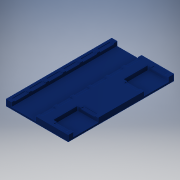
# Autodesk Inventor part: Assembly Plate
Saved by Autodesk Inventor 2019.4 (Build 234330000, 330)
## iProperties
Created: 2021-01-11
Part Number: Assembly Plate
Material: Aluminum, Anodized Blue
Document SubType Name: Modeling
Designer: caleb
Density: 2.7 g/cm^3
Appearance: Anodized - Blue
Author: caleb
Autodesk Inventor part; units mm, degrees
ref_plane "YZ Plane" through (0, 0, 0) normal (1, 0, 0) x (0, 1, 0)
ref_plane "XZ Plane" through (0, 0, 0) normal (0, 1, 0) x (-1, 0, 0)
ref_plane "XY Plane" through (0, 0, 0) normal (0, 0, 1) x (1, 0, 0)
sketch "Sketch1" plane through (0, 0, 0) normal (0, 1, 0) x (-1, 0, 0)
  line L0 (-63.5, 107.95) -> (63.5, 107.95)
  line L1 (63.5, 107.95) -> (63.5, -107.95)
  line L2 (63.5, -107.95) -> (-63.5, -107.95)
  line L3 (-63.5, -107.95) -> (-63.5, 107.95)
  line L4 (-63.5, 107.95) -> (63.5, -107.95) construction
  line L5 (63.5, 107.95) -> (-63.5, -107.95) construction
  point P0 (0, 0)
  dimension "d0" = 127
  dimension "d1" = 215.9
  constraints: 12 end point, 2 midpoint, 2 parallel, 1 horizontal, 1 perpendicular
  measures "d0" distance of L1.end L2.end
  measures "d1" distance of L0.end L1.end
extrude "Extrusion1" add sketch "Sketch1" along normal blind 12.7
sketch "Sketch8" plane through (0, 12.7, 0) normal (0, 1, 0) x (1, 0, 0)
  line L0 (-63.5, -107.95) -> (63.5, -107.95) projected
  line L1 (63.5, 107.95) -> (-63.5, 107.95) projected
  line L2 (-63.5, 107.95) -> (-63.5, -107.95) projected
  line L3 (63.5, -107.95) -> (63.5, 107.95) projected
  line L4 (-52.5, -107.95) -> (-2.5, -107.95)
  line L5 (-2.5, -107.95) -> (-2.5, 107.95)
  line L6 (-2.5, 107.95) -> (-52.5, 107.95)
  line L7 (-52.5, 107.95) -> (-52.5, -107.95)
  point P0 (0, 0)
  dimension "d91" = 11
  dimension "d92" = 50
  constraints: 8 end point, 2 parallel, 2 point on line, 1 horizontal, 1 perpendicular
  measures "d91" distance between parallel lines of L2 L7
  measures "d92" distance between parallel lines of L7 L5
extrude "Extrusion7" cut sketch "Sketch8" against normal blind 9 contours L7 L1 L5 L0
sketch "Sketch9" plane through (0, 12.7, 0) normal (0, 1, 0) x (1, 0, 0)
  line L0 (-63.5, -107.95) -> (-52.5, -107.95) projected
  line L1 (-63.5, 107.95) -> (-63.5, -107.95) projected
  line L2 (-52.5, -107.95) -> (-52.5, 107.95) projected
  line L3 (-52.5, -100.922) -> (-59, -100.922)
  line L4 (-59, -100.922) -> (-59, -74.122)
  line L5 (-58, -73.122) -> (-52.5, -73.122)
  line L6 (-52.5, -73.122) -> (-52.5, -100.922)
  circle A0 centre (-59, -100.922) radius 1
  line L7 (-2.5, 107.95) -> (-2.5, -107.95) projected
  line L8 (-2.5, -107.95) -> (63.5, -107.95) projected
  line L9 (-2.5, -100.922) -> (3, -100.922)
  line L10 (4, -99.922) -> (4, -74.122)
  line L11 (3, -73.122) -> (-2.5, -73.122)
  line L12 (-2.5, -73.122) -> (-2.5, -100.922)
  arc A1 (-58, -73.122) -> (-59, -74.122) centre (-58, -74.122) ccw
  arc A2 (4, -74.122) -> (3, -73.122) centre (3, -74.122) ccw
  arc A3 (3, -100.922) -> (4, -99.922) centre (3, -99.922) ccw
  arc A4 (4, -39.294) -> (3, -38.294) centre (3, -39.294) ccw
  line L13 (-2.5, -38.294) -> (-2.5, -66.094)
  line L14 (4, -65.094) -> (4, -39.294)
  line L15 (-2.5, -66.094) -> (3, -66.094)
  arc A5 (3, -66.094) -> (4, -65.094) centre (3, -65.094) ccw
  line L16 (3, -38.294) -> (-2.5, -38.294)
  line L17 (-52.5, -38.294) -> (-52.5, -66.094)
  line L18 (-58, -38.294) -> (-52.5, -38.294)
  arc A6 (-58, -38.294) -> (-59, -39.294) centre (-58, -39.294) ccw
  line L19 (-59, -66.094) -> (-59, -39.294)
  line L20 (-52.5, -66.094) -> (-59, -66.094)
  circle A7 centre (-59, -66.094) radius 1
  arc A8 (4, -4.466) -> (3, -3.466) centre (3, -4.466) ccw
  line L21 (-2.5, -3.466) -> (-2.5, -31.266)
  line L22 (4, -30.266) -> (4, -4.466)
  line L23 (-2.5, -31.266) -> (3, -31.266)
  arc A9 (3, -31.266) -> (4, -30.266) centre (3, -30.266) ccw
  line L24 (3, -3.466) -> (-2.5, -3.466)
  line L25 (-52.5, -3.466) -> (-52.5, -31.266)
  line L26 (-58, -3.466) -> (-52.5, -3.466)
  arc A10 (-58, -3.466) -> (-59, -4.466) centre (-58, -4.466) ccw
  line L27 (-59, -31.266) -> (-59, -4.466)
  line L28 (-52.5, -31.266) -> (-59, -31.266)
  circle A11 centre (-59, -31.266) radius 1
  arc A12 (4, 30.362) -> (3, 31.362) centre (3, 30.362) ccw
  line L29 (-2.5, 31.362) -> (-2.5, 3.562)
  line L30 (4, 4.562) -> (4, 30.362)
  line L31 (-2.5, 3.562) -> (3, 3.562)
  arc A13 (3, 3.562) -> (4, 4.562) centre (3, 4.562) ccw
  line L32 (3, 31.362) -> (-2.5, 31.362)
  line L33 (-52.5, 31.362) -> (-52.5, 3.562)
  line L34 (-58, 31.362) -> (-52.5, 31.362)
  arc A14 (-58, 31.362) -> (-59, 30.362) centre (-58, 30.362) ccw
  line L35 (-59, 3.562) -> (-59, 30.362)
  line L36 (-52.5, 3.562) -> (-59, 3.562)
  circle A15 centre (-59, 3.562) radius 1
  arc A16 (4, 65.19) -> (3, 66.19) centre (3, 65.19) ccw
  line L37 (-2.5, 66.19) -> (-2.5, 38.39)
  line L38 (4, 39.39) -> (4, 65.19)
  line L39 (-2.5, 38.39) -> (3, 38.39)
  arc A17 (3, 38.39) -> (4, 39.39) centre (3, 39.39) ccw
  line L40 (3, 66.19) -> (-2.5, 66.19)
  line L41 (-52.5, 66.19) -> (-52.5, 38.39)
  line L42 (-58, 66.19) -> (-52.5, 66.19)
  arc A18 (-58, 66.19) -> (-59, 65.19) centre (-58, 65.19) ccw
  line L43 (-59, 38.39) -> (-59, 65.19)
  line L44 (-52.5, 38.39) -> (-59, 38.39)
  circle A19 centre (-59, 38.39) radius 1
  arc A20 (4, 100.018) -> (3, 101.018) centre (3, 100.018) ccw
  line L45 (-2.5, 101.018) -> (-2.5, 73.218)
  line L46 (4, 74.218) -> (4, 100.018)
  line L47 (-2.5, 73.218) -> (3, 73.218)
  arc A21 (3, 73.218) -> (4, 74.218) centre (3, 74.218) ccw
  line L48 (3, 101.018) -> (-2.5, 101.018)
  line L49 (-52.5, 101.018) -> (-52.5, 73.218)
  line L50 (-58, 101.018) -> (-52.5, 101.018)
  arc A22 (-58, 101.018) -> (-59, 100.018) centre (-58, 100.018) ccw
  line L51 (-59, 73.218) -> (-59, 100.018)
  line L52 (-52.5, 73.218) -> (-59, 73.218)
  circle A23 centre (-59, 73.218) radius 1
  point P0 (0, 0)
  point P1 (-59, -73.122)
  point P2 (4, -73.122)
  point P3 (4, -100.922)
  point P4 (4, -38.294)
  point P5 (4, -66.094)
  point P6 (-59, -38.294)
  point P7 (4, -3.466)
  point P8 (4, -31.266)
  point P9 (-59, -3.466)
  point P10 (4, 31.362)
  point P11 (4, 3.562)
  point P12 (-59, 31.362)
  point P13 (4, 66.19)
  point P14 (4, 38.39)
  point P15 (-59, 66.19)
  point P16 (4, 101.018)
  point P17 (4, 73.218)
  point P18 (-59, 101.018)
  dimension "d95" = 7.028
  dimension "d96" = 27.8
  dimension "d97" = 2
  dimension "d99" = 6.5
  dimension "d100" = 7.028
  dimension "d101" = 27.8
  dimension "d102" = 6.5
  dimension "d105" = 1
  dimension "d108" = 34.828
  constraints: 96 end point, 38 point on line, 36 point on circle, 24 centre point, 6 coincident, 6 tangent, 4 parallel, 2 equal radius, 2 horizontal, 2 perpendicular, 1 vertical, 150 other
  measures "d95" distance between parallel lines of L0 L3
  measures "d96" distance of L3.end point (-59, -73.122)
  measures "d97" diameter of A0
  measures "d99" distance of L3.start L3.end
  measures "d100" distance between parallel lines of L8 L9
  measures "d101" distance of point (4, -100.922) point (4, -73.122)
  measures "d102" distance of point (4, -73.122) L11.end
  measures "d105" radius of A1
  measures "d108" distance of L11.end L13.start
extrude "Extrusion8" cut sketch "Sketch9" against normal blind 2
sketch "Sketch10" plane through (0, 12.7, 0) normal (0, 1, 0) x (1, 0, 0)
  line L0 (63.5, 107.95) -> (63.5, -107.95) projected
  line L1 (63.5, -96.95) -> (22.5, -96.95)
  line L2 (21.5, -95.95) -> (21.5, -47.95)
  line L3 (22.5, -46.95) -> (63.5, -46.95)
  line L4 (63.5, -46.95) -> (63.5, -96.95)
  line L5 (-2.5, -107.95) -> (63.5, -107.95) projected
  line L6 (56.472, -96.95) -> (28.672, -96.95)
  line L7 (28.672, -96.95) -> (28.672, -102.45)
  line L8 (29.672, -103.45) -> (56.472, -103.45)
  line L9 (56.472, -103.45) -> (56.472, -96.95)
  line L10 (56.472, -46.95) -> (28.672, -46.95)
  line L11 (28.672, -46.95) -> (28.672, -41.45)
  line L12 (29.672, -40.45) -> (55.472, -40.45)
  line L13 (56.472, -41.45) -> (56.472, -46.95)
  circle A0 centre (56.472, -103.45) radius 1
  arc A1 (28.672, -102.45) -> (29.672, -103.45) centre (29.672, -102.45) ccw
  arc A2 (29.672, -40.45) -> (28.672, -41.45) centre (29.672, -41.45) ccw
  arc A3 (56.472, -41.45) -> (55.472, -40.45) centre (55.472, -41.45) ccw
  arc A4 (22.5, -46.95) -> (21.5, -47.95) centre (22.5, -47.95) ccw
  arc A5 (21.5, -95.95) -> (22.5, -96.95) centre (22.5, -95.95) ccw
  line L14 (63.5, 0) -> (16.2003, 0)
  line L15 (63.5, -107.95) -> (63.5, 107.95)
  line L16 (63.5, 96.95) -> (22.5, 96.95)
  line L17 (21.5, 95.95) -> (21.5, 47.95)
  line L18 (22.5, 46.95) -> (63.5, 46.95)
  line L19 (63.5, 46.95) -> (63.5, 96.95)
  line L20 (56.472, 96.95) -> (28.672, 96.95)
  line L21 (28.672, 96.95) -> (28.672, 102.45)
  line L22 (29.672, 103.45) -> (56.472, 103.45)
  line L23 (56.472, 103.45) -> (56.472, 96.95)
  line L24 (56.472, 46.95) -> (28.672, 46.95)
  line L25 (28.672, 46.95) -> (28.672, 41.45)
  line L26 (29.672, 40.45) -> (55.472, 40.45)
  line L27 (56.472, 41.45) -> (56.472, 46.95)
  circle A6 centre (56.472, 103.45) radius 1
  arc A7 (29.672, 103.45) -> (28.672, 102.45) centre (29.672, 102.45) ccw
  arc A8 (28.672, 41.45) -> (29.672, 40.45) centre (29.672, 41.45) ccw
  arc A9 (55.472, 40.45) -> (56.472, 41.45) centre (55.472, 41.45) ccw
  arc A10 (21.5, 47.95) -> (22.5, 46.95) centre (22.5, 47.95) ccw
  arc A11 (22.5, 96.95) -> (21.5, 95.95) centre (22.5, 95.95) ccw
  point P0 (0, 0)
  point P1 (21.5, -46.95)
  point P2 (21.5, -96.95)
  point P3 (28.672, -103.45)
  point P4 (28.672, -40.45)
  point P5 (56.472, -40.45)
  point P6 (21.5, 46.95)
  point P7 (21.5, 96.95)
  point P8 (28.672, 103.45)
  point P9 (28.672, 40.45)
  point P10 (56.472, 40.45)
  dimension "d115" = 50
  dimension "d116" = 11
  dimension "d117" = 42
  dimension "d118" = 7.028
  dimension "d119" = 27.8
  dimension "d120" = 6.5
  dimension "d121" = 6.5
  dimension "d122" = 7.028
  dimension "d123" = 27.8
  dimension "d124" = 2
  dimension "d125" = 1
  constraints: 52 end point, 30 symmetric about line, 26 point on line, 20 point on circle, 12 centre point, 10 tangent, 6 parallel, 4 equal radius, 4 horizontal, 3 perpendicular, 2 coincident, 1 midpoint, 6 other
  measures "d115" distance of point (21.5, -96.95) point (21.5, -46.95)
  measures "d116" distance between parallel lines of L5 L1
  measures "d117" distance of L1.start point (21.5, -96.95)
  measures "d118" distance between parallel lines of L0 L9
  measures "d119" distance of point (28.672, -103.45) L8.end
  measures "d120" distance between parallel lines of L8 L6
  measures "d121" distance of L10.end point (28.672, -40.45)
  measures "d122" distance between parallel lines of L0 L13
  measures "d123" distance of point (28.672, -40.45) point (56.472, -40.45)
  measures "d124" diameter of A0
  measures "d125" radius of A1
extrude "Extrusion9" cut sketch "Sketch10" against normal blind 9 contours L0 L18 A10 L17 A11 L16 | L0 L1 A5 L2 A4 L3
extrude "Extrusion10" cut sketch "Sketch10" against normal blind 2 contours L16 L21 A7 L22 A6 L23 | L27 A9 L26 A8 L25 L18 | A6 L22 L23 | L23 L22 A6 | L3 L11 A2 L12 A3 L13 | L9 A0 L8 A1 L7 L1 | A0 L8 L9 | L9 L8 A0
body "Solid1"
